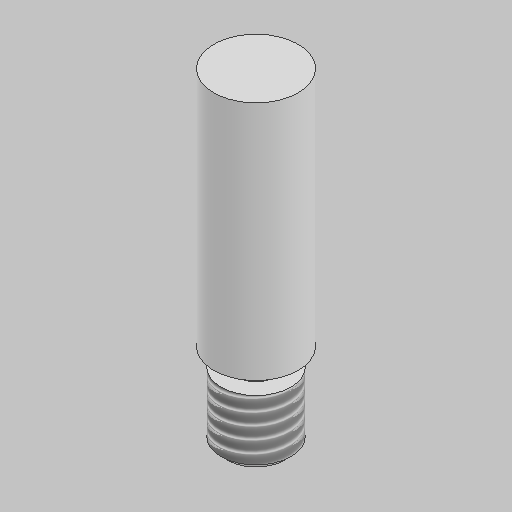
# Autodesk Inventor part: HeatBreak
Saved by Autodesk Inventor 2025.4 (Build 294407000, 407)
## iProperties
Created: 2026-03-02
Part Number: HeatBreak
Material: Genérico
Document SubType Name: Modeling
Designer: Inema
Density: 1 g/cm^3
Appearance: Valor por defecto
Author: Inema
Autodesk Inventor part; units mm, degrees
ref_plane "YZ Plane" through (0, 0, 0) normal (1, 0, 0) x (0, 1, 0)
ref_plane "XZ Plane" through (0, 0, 0) normal (0, 1, 0) x (-1, 0, 0)
ref_plane "XY Plane" through (0, 0, 0) normal (0, 0, 1) x (1, 0, 0)
sketch "Boceto1" plane through (0, 0, 0) normal (0, 0, 1) x (1, 0, 0)
  line L0 (0, 6.1211) -> (0, -20.8789)
  line L1 (0, -20.8789) -> (2.9, -20.8789)
  line L2 (2.9, -20.8789) -> (2.9, -15.3789)
  line L3 (2.9, -15.3789) -> (1.5, -15.3789)
  line L4 (1.5, -15.3789) -> (1.5, -13.8789)
  line L5 (1.5, -13.8789) -> (3.5, -13.8789)
  line L6 (3.5, -13.8789) -> (3.5, 6.1211)
  line L7 (3.5, 6.1211) -> (0, 6.1211)
  point P0 (0, 0)
  point P1 (1.45, -20.8789)
  point P2 (1.5, -14.6289)
  dimension "d0" = 3.5
  dimension "d1" = 20
  dimension "d2" = 27
  dimension "d3" = 5.5
  dimension "d4" = 2.9
  dimension "d5" = 1.5
  constraints: 16 end point, 7 perpendicular, 2 midpoint, 1 vertical
  measures "d0" distance of L6.end L0.start
  measures "d1" distance of L5.end L6.end
  measures "d2" vertical distance of L6.end point (1.45, -20.879)
  measures "d3" distance of L1.end L2.end
  measures "d4" distance of L0.end L1.end
  measures "d5" distance from line of L0 point (1.5, -14.629)
revolve "Revolución1" add sketch "Boceto1" angle 360 about axis through (0, 6.1211, 0) along (0, -1, 0)
chamfer "Chaflán1" distance 0.5 angle 45 1 edges at (-2.9, -20.8789, 0)
thread "Rosca1" size "M6x1" class "6g" standard "ANSI Metric M Profile" full length
